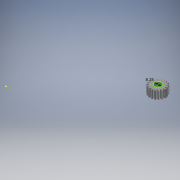
# Autodesk Inventor part: gear_z18_m1
Saved by Autodesk Inventor 2019 (Build 230136000, 136)
## iProperties
Created: 2015-11-26
Part Number: gear_z18_m1
Document SubType Name: Modeling
Designer: VozarikL
Material: Generic
Density: 1 g/cm^3
Appearance: Aluminum - Polished
Autodesk Inventor part; units mm, degrees
ref_plane "YZ Plane" through (0, 0, 0) normal (1, 0, 0) x (0, 1, 0)
ref_plane "XZ Plane" through (0, 0, 0) normal (0, 1, 0) x (-1, 0, 0)
ref_plane "XY Plane" through (0, 0, 0) normal (0, 0, 1) x (1, 0, 0)
sketch "Vázlat1" plane through (0, 0, 0) normal (0, 0, 1) x (1, 0, 0)
  arc A0 (98.9683, 94.0647) -> (99.0231, 94.4245) centre (91.2444, 95.4266) ccw
  arc A1 (99.2517, 94.6057) -> (99.0231, 94.4245) centre (99.2304, 94.3977) ccw
  line L0 (99.2517, 94.6057) -> (99.6575, 94.564)
  line L1 (99.6575, 94.564) -> (99.6743, 94.563)
  line L2 (99.6743, 94.563) -> (99.7248, 94.5628)
  line L3 (99.7248, 94.5628) -> (99.8089, 94.5677)
  line L4 (99.8089, 94.5677) -> (99.9258, 94.5818)
  line L5 (99.9258, 94.5818) -> (100.0748, 94.6094)
  line L6 (100.0748, 94.6094) -> (100.2544, 94.6544)
  line L7 (100.2544, 94.6544) -> (100.4629, 94.7209)
  line L8 (100.4629, 94.7209) -> (100.6981, 94.8126)
  line L9 (100.6981, 94.8126) -> (100.9576, 94.9332)
  line L10 (100.9576, 94.9332) -> (101.2386, 95.0859)
  arc A2 (101.2386, 95.0859) -> (101.2444, 95.4266) centre (91.2444, 95.4266) ccw
  arc A3 (99.0231, 96.4288) -> (98.9683, 96.7885) centre (91.2444, 95.4266) ccw
  arc A4 (99.0231, 96.4288) -> (99.2517, 96.2476) centre (99.2304, 96.4555) ccw
  line L11 (99.2517, 96.2476) -> (99.6575, 96.2892)
  line L12 (99.6575, 96.2892) -> (99.6743, 96.2902)
  line L13 (99.6743, 96.2902) -> (99.7248, 96.2904)
  line L14 (99.7248, 96.2904) -> (99.8089, 96.2856)
  line L15 (99.8089, 96.2856) -> (99.9258, 96.2714)
  line L16 (99.9258, 96.2714) -> (100.0748, 96.2439)
  line L17 (100.0748, 96.2439) -> (100.2544, 96.1988)
  line L18 (100.2544, 96.1988) -> (100.4629, 96.1323)
  line L19 (100.4629, 96.1323) -> (100.6981, 96.0406)
  line L20 (100.6981, 96.0406) -> (100.9576, 95.9201)
  line L21 (100.9576, 95.9201) -> (101.2386, 95.7674)
  arc A5 (101.2444, 95.4266) -> (101.2386, 95.7674) centre (91.2444, 95.4266) ccw
  arc A6 (98.9683, 96.7885) -> (98.8968, 97.1454) centre (91.2444, 95.4266) ccw
  arc A7 (99.0496, 97.3938) -> (98.8968, 97.1454) centre (99.1007, 97.1912) ccw
  line L22 (99.0496, 97.3938) -> (99.4452, 97.4935)
  line L23 (99.4452, 97.4935) -> (99.4613, 97.4983)
  line L24 (99.4613, 97.4983) -> (99.5088, 97.5154)
  line L25 (99.5088, 97.5154) -> (99.5861, 97.5487)
  line L26 (99.5861, 97.5487) -> (99.6912, 97.602)
  line L27 (99.6912, 97.602) -> (99.8218, 97.6788)
  line L28 (99.8218, 97.6788) -> (99.9751, 97.7826)
  line L29 (99.9751, 97.7826) -> (100.1483, 97.9164)
  line L30 (100.1483, 97.9164) -> (100.338, 98.083)
  line L31 (100.338, 98.083) -> (100.5406, 98.285)
  line L32 (100.5406, 98.285) -> (100.7524, 98.5246)
  arc A8 (100.7524, 98.5246) -> (100.6413, 98.8468) centre (91.2444, 95.4266) ccw
  arc A9 (98.2112, 99.0288) -> (98.0366, 99.3481) centre (91.2444, 95.4266) ccw
  arc A10 (98.2112, 99.0288) -> (98.488, 98.9368) centre (98.3969, 99.1248) ccw
  line L33 (98.488, 98.9368) -> (98.8551, 99.1146)
  line L34 (98.8551, 99.1146) -> (98.8706, 99.1213)
  line L35 (98.8706, 99.1213) -> (98.918, 99.1388)
  line L36 (98.918, 99.1388) -> (98.9986, 99.163)
  line L37 (98.9986, 99.163) -> (99.1133, 99.1897)
  line L38 (99.1133, 99.1897) -> (99.2627, 99.2148)
  line L39 (99.2627, 99.2148) -> (99.4469, 99.2339)
  line L40 (99.4469, 99.2339) -> (99.6655, 99.2427)
  line L41 (99.6655, 99.2427) -> (99.918, 99.2369)
  line L42 (99.918, 99.2369) -> (100.2031, 99.2124)
  line L43 (100.2031, 99.2124) -> (100.5193, 99.1651)
  arc A11 (100.6413, 98.8468) -> (100.5193, 99.1651) centre (91.2444, 95.4266) ccw
  arc A12 (98.0366, 99.3481) -> (97.8474, 99.659) centre (91.2444, 95.4266) ccw
  arc A13 (97.9061, 99.9447) -> (97.8474, 99.659) centre (98.0234, 99.7718) ccw
  line L44 (97.9061, 99.9447) -> (98.2437, 100.1737)
  line L45 (98.2437, 100.1737) -> (98.2572, 100.1837)
  line L46 (98.2572, 100.1837) -> (98.296, 100.216)
  line L47 (98.296, 100.216) -> (98.3573, 100.2738)
  line L48 (98.3573, 100.2738) -> (98.4378, 100.3598)
  line L49 (98.4378, 100.3598) -> (98.5342, 100.4766)
  line L50 (98.5342, 100.4766) -> (98.6428, 100.6266)
  line L51 (98.6428, 100.6266) -> (98.7598, 100.8115)
  line L52 (98.7598, 100.8115) -> (98.881, 101.033)
  line L53 (98.881, 101.033) -> (99.0023, 101.2921)
  line L54 (99.0023, 101.2921) -> (99.1194, 101.5897)
  arc A14 (99.1194, 101.5897) -> (98.9049, 101.8545) centre (91.2444, 95.4266) ccw
  arc A15 (96.5591, 101.1944) -> (96.2858, 101.4347) centre (91.2444, 95.4266) ccw
  arc A16 (96.5591, 101.1944) -> (96.8507, 101.2025) centre (96.7007, 101.3481) ccw
  line L55 (96.8507, 101.2025) -> (97.1348, 101.4953)
  line L56 (97.1348, 101.4953) -> (97.147, 101.5068)
  line L57 (97.147, 101.5068) -> (97.1856, 101.5394)
  line L58 (97.1856, 101.5394) -> (97.253, 101.5897)
  line L59 (97.253, 101.5897) -> (97.3517, 101.6541)
  line L60 (97.3517, 101.6541) -> (97.4836, 101.7287)
  line L61 (97.4836, 101.7287) -> (97.6501, 101.8097)
  line L62 (97.6501, 101.8097) -> (97.8525, 101.8927)
  line L63 (97.8525, 101.8927) -> (98.0917, 101.9737)
  line L64 (98.0917, 101.9737) -> (98.368, 102.0482)
  line L65 (98.368, 102.0482) -> (98.6814, 102.1118)
  arc A17 (98.9049, 101.8545) -> (98.6814, 102.1118) centre (91.2444, 95.4266) ccw
  arc A18 (96.2858, 101.4347) -> (96.0017, 101.6621) centre (91.2444, 95.4266) ccw
  arc A19 (95.959, 101.9507) -> (96.0017, 101.6621) centre (96.1284, 101.8283) ccw
  line L66 (95.959, 101.9507) -> (96.198, 102.2813)
  line L67 (96.198, 102.2813) -> (96.2073, 102.2954)
  line L68 (96.2073, 102.2954) -> (96.2327, 102.339)
  line L69 (96.2327, 102.339) -> (96.2705, 102.4142)
  line L70 (96.2705, 102.4142) -> (96.3168, 102.5226)
  line L71 (96.3168, 102.5226) -> (96.3674, 102.6653)
  line L72 (96.3674, 102.6653) -> (96.4181, 102.8434)
  line L73 (96.4181, 102.8434) -> (96.4648, 103.0572)
  line L74 (96.4648, 103.0572) -> (96.503, 103.3068)
  line L75 (96.503, 103.3068) -> (96.5284, 103.5918)
  line L76 (96.5284, 103.5918) -> (96.5366, 103.9115)
  arc A20 (96.5366, 103.9115) -> (96.2444, 104.0869) centre (91.2444, 95.4266) ccw
  arc A21 (94.2659, 102.6643) -> (93.9269, 102.7966) centre (91.2444, 95.4266) ccw
  arc A22 (94.2659, 102.6643) -> (94.5371, 102.7716) centre (94.3464, 102.8571) ccw
  line L77 (94.5371, 102.7716) -> (94.704, 103.1439)
  line L78 (94.704, 103.1439) -> (94.7115, 103.159)
  line L79 (94.7115, 103.159) -> (94.7366, 103.2028)
  line L80 (94.7366, 103.2028) -> (94.7828, 103.2731)
  line L81 (94.7828, 103.2731) -> (94.8535, 103.3674)
  line L82 (94.8535, 103.3674) -> (94.9518, 103.4826)
  line L83 (94.9518, 103.4826) -> (95.0806, 103.6156)
  line L84 (95.0806, 103.6156) -> (95.2425, 103.7629)
  line L85 (95.2425, 103.7629) -> (95.4395, 103.9207)
  line L86 (95.4395, 103.9207) -> (95.6737, 104.0852)
  line L87 (95.6737, 104.0852) -> (95.9464, 104.2522)
  arc A23 (96.2444, 104.0869) -> (95.9464, 104.2522) centre (91.2444, 95.4266) ccw
  arc A24 (93.9269, 102.7966) -> (93.5821, 102.9131) centre (91.2444, 95.4266) ccw
  arc A25 (93.4434, 103.1697) -> (93.5821, 102.9131) centre (93.6444, 103.1126) ccw
  line L88 (93.4434, 103.1697) -> (93.5548, 103.5622)
  line L89 (93.5548, 103.5622) -> (93.5587, 103.5785)
  line L90 (93.5587, 103.5785) -> (93.5677, 103.6282)
  line L91 (93.5677, 103.6282) -> (93.5775, 103.7118)
  line L92 (93.5775, 103.7118) -> (93.5839, 103.8295)
  line L93 (93.5839, 103.8295) -> (93.5826, 103.9809)
  line L94 (93.5826, 103.9809) -> (93.5694, 104.1656)
  line L95 (93.5694, 104.1656) -> (93.5402, 104.3825)
  line L96 (93.5402, 104.3825) -> (93.4907, 104.6301)
  line L97 (93.4907, 104.6301) -> (93.4171, 104.9066)
  line L98 (93.4171, 104.9066) -> (93.3155, 105.2098)
  arc A26 (93.3155, 105.2098) -> (92.9809, 105.2747) centre (91.2444, 95.4266) ccw
  arc A27 (91.6082, 103.2612) -> (91.2444, 103.2696) centre (91.2444, 95.4266) ccw
  arc A28 (91.6082, 103.2612) -> (91.8264, 103.4548) centre (91.6179, 103.47) ccw
  line L99 (91.8264, 103.4548) -> (91.8559, 103.8617)
  line L100 (91.8559, 103.8617) -> (91.8578, 103.8785)
  line L101 (91.8578, 103.8785) -> (91.8664, 103.9282)
  line L102 (91.8664, 103.9282) -> (91.8857, 104.0101)
  line L103 (91.8857, 104.0101) -> (91.9199, 104.1229)
  line L104 (91.9199, 104.1229) -> (91.9729, 104.2648)
  line L105 (91.9729, 104.2648) -> (92.0485, 104.4338)
  line L106 (92.0485, 104.4338) -> (92.1502, 104.6276)
  line L107 (92.1502, 104.6276) -> (92.2814, 104.8433)
  line L108 (92.2814, 104.8433) -> (92.4451, 105.0779)
  line L109 (92.4451, 105.0779) -> (92.6443, 105.3282)
  arc A29 (92.9809, 105.2747) -> (92.6443, 105.3282) centre (91.2444, 95.4266) ccw
  arc A30 (91.2444, 103.2696) -> (90.8806, 103.2612) centre (91.2444, 95.4266) ccw
  arc A31 (90.6625, 103.4548) -> (90.8806, 103.2612) centre (90.8709, 103.47) ccw
  line L110 (90.6625, 103.4548) -> (90.633, 103.8617)
  line L111 (90.633, 103.8617) -> (90.631, 103.8785)
  line L112 (90.631, 103.8785) -> (90.6225, 103.9282)
  line L113 (90.6225, 103.9282) -> (90.6031, 104.0101)
  line L114 (90.6031, 104.0101) -> (90.5689, 104.1229)
  line L115 (90.5689, 104.1229) -> (90.5159, 104.2648)
  line L116 (90.5159, 104.2648) -> (90.4403, 104.4338)
  line L117 (90.4403, 104.4338) -> (90.3386, 104.6276)
  line L118 (90.3386, 104.6276) -> (90.2075, 104.8433)
  line L119 (90.2075, 104.8433) -> (90.0437, 105.0779)
  line L120 (90.0437, 105.0779) -> (89.8445, 105.3282)
  arc A32 (89.8445, 105.3282) -> (89.5079, 105.2747) centre (91.2444, 95.4266) ccw
  arc A33 (88.9067, 102.9131) -> (88.5619, 102.7966) centre (91.2444, 95.4266) ccw
  arc A34 (88.9067, 102.9131) -> (89.0455, 103.1697) centre (88.8444, 103.1126) ccw
  line L121 (89.0455, 103.1697) -> (88.934, 103.5622)
  line L122 (88.934, 103.5622) -> (88.9301, 103.5785)
  line L123 (88.9301, 103.5785) -> (88.9211, 103.6282)
  line L124 (88.9211, 103.6282) -> (88.9113, 103.7118)
  line L125 (88.9113, 103.7118) -> (88.9049, 103.8295)
  line L126 (88.9049, 103.8295) -> (88.9062, 103.9809)
  line L127 (88.9062, 103.9809) -> (88.9194, 104.1656)
  line L128 (88.9194, 104.1656) -> (88.9487, 104.3825)
  line L129 (88.9487, 104.3825) -> (88.9981, 104.6301)
  line L130 (88.9981, 104.6301) -> (89.0718, 104.9066)
  line L131 (89.0718, 104.9066) -> (89.1733, 105.2098)
  arc A35 (89.5079, 105.2747) -> (89.1733, 105.2098) centre (91.2444, 95.4266) ccw
  arc A36 (88.5619, 102.7966) -> (88.223, 102.6643) centre (91.2444, 95.4266) ccw
  arc A37 (87.9517, 102.7716) -> (88.223, 102.6643) centre (88.1425, 102.8571) ccw
  line L132 (87.9517, 102.7716) -> (87.7849, 103.1439)
  line L133 (87.7849, 103.1439) -> (87.7773, 103.159)
  line L134 (87.7773, 103.159) -> (87.7523, 103.2028)
  line L135 (87.7523, 103.2028) -> (87.7061, 103.2731)
  line L136 (87.7061, 103.2731) -> (87.6353, 103.3674)
  line L137 (87.6353, 103.3674) -> (87.537, 103.4826)
  line L138 (87.537, 103.4826) -> (87.4082, 103.6156)
  line L139 (87.4082, 103.6156) -> (87.2464, 103.7629)
  line L140 (87.2464, 103.7629) -> (87.0493, 103.9207)
  line L141 (87.0493, 103.9207) -> (86.8152, 104.0852)
  line L142 (86.8152, 104.0852) -> (86.5424, 104.2522)
  arc A38 (86.5424, 104.2522) -> (86.2444, 104.0869) centre (91.2444, 95.4266) ccw
  arc A39 (86.4871, 101.6621) -> (86.203, 101.4347) centre (91.2444, 95.4266) ccw
  arc A40 (86.4871, 101.6621) -> (86.5298, 101.9507) centre (86.3604, 101.8283) ccw
  line L143 (86.5298, 101.9507) -> (86.2908, 102.2813)
  line L144 (86.2908, 102.2813) -> (86.2816, 102.2954)
  line L145 (86.2816, 102.2954) -> (86.2561, 102.339)
  line L146 (86.2561, 102.339) -> (86.2183, 102.4142)
  line L147 (86.2183, 102.4142) -> (86.1721, 102.5226)
  line L148 (86.1721, 102.5226) -> (86.1215, 102.6653)
  line L149 (86.1215, 102.6653) -> (86.0707, 102.8434)
  line L150 (86.0707, 102.8434) -> (86.024, 103.0572)
  line L151 (86.024, 103.0572) -> (85.9858, 103.3068)
  line L152 (85.9858, 103.3068) -> (85.9605, 103.5918)
  line L153 (85.9605, 103.5918) -> (85.9522, 103.9115)
  arc A41 (86.2444, 104.0869) -> (85.9522, 103.9115) centre (91.2444, 95.4266) ccw
  arc A42 (86.203, 101.4347) -> (85.9298, 101.1944) centre (91.2444, 95.4266) ccw
  arc A43 (85.6382, 101.2025) -> (85.9298, 101.1944) centre (85.7881, 101.3481) ccw
  line L154 (85.6382, 101.2025) -> (85.354, 101.4953)
  line L155 (85.354, 101.4953) -> (85.3418, 101.5068)
  line L156 (85.3418, 101.5068) -> (85.3033, 101.5394)
  line L157 (85.3033, 101.5394) -> (85.2358, 101.5897)
  line L158 (85.2358, 101.5897) -> (85.1371, 101.6541)
  line L159 (85.1371, 101.6541) -> (85.0053, 101.7287)
  line L160 (85.0053, 101.7287) -> (84.8387, 101.8097)
  line L161 (84.8387, 101.8097) -> (84.6363, 101.8927)
  line L162 (84.6363, 101.8927) -> (84.3971, 101.9737)
  line L163 (84.3971, 101.9737) -> (84.1209, 102.0482)
  line L164 (84.1209, 102.0482) -> (83.8075, 102.1118)
  arc A44 (83.8075, 102.1118) -> (83.584, 101.8545) centre (91.2444, 95.4266) ccw
  arc A45 (84.6414, 99.659) -> (84.4522, 99.3481) centre (91.2444, 95.4266) ccw
  arc A46 (84.6414, 99.659) -> (84.5827, 99.9447) centre (84.4654, 99.7718) ccw
  line L165 (84.5827, 99.9447) -> (84.2451, 100.1737)
  line L166 (84.2451, 100.1737) -> (84.2316, 100.1837)
  line L167 (84.2316, 100.1837) -> (84.1928, 100.216)
  line L168 (84.1928, 100.216) -> (84.1315, 100.2738)
  line L169 (84.1315, 100.2738) -> (84.051, 100.3598)
  line L170 (84.051, 100.3598) -> (83.9546, 100.4766)
  line L171 (83.9546, 100.4766) -> (83.846, 100.6266)
  line L172 (83.846, 100.6266) -> (83.7291, 100.8115)
  line L173 (83.7291, 100.8115) -> (83.6078, 101.033)
  line L174 (83.6078, 101.033) -> (83.4865, 101.2921)
  line L175 (83.4865, 101.2921) -> (83.3694, 101.5897)
  arc A47 (83.584, 101.8545) -> (83.3694, 101.5897) centre (91.2444, 95.4266) ccw
  arc A48 (84.4522, 99.3481) -> (84.2776, 99.0288) centre (91.2444, 95.4266) ccw
  arc A49 (84.0008, 98.9368) -> (84.2776, 99.0288) centre (84.0919, 99.1248) ccw
  line L176 (84.0008, 98.9368) -> (83.6337, 99.1146)
  line L177 (83.6337, 99.1146) -> (83.6182, 99.1213)
  line L178 (83.6182, 99.1213) -> (83.5709, 99.1388)
  line L179 (83.5709, 99.1388) -> (83.4902, 99.163)
  line L180 (83.4902, 99.163) -> (83.3755, 99.1897)
  line L181 (83.3755, 99.1897) -> (83.2261, 99.2148)
  line L182 (83.2261, 99.2148) -> (83.0419, 99.2339)
  line L183 (83.0419, 99.2339) -> (82.8233, 99.2427)
  line L184 (82.8233, 99.2427) -> (82.5709, 99.2369)
  line L185 (82.5709, 99.2369) -> (82.2858, 99.2124)
  line L186 (82.2858, 99.2124) -> (81.9695, 99.1651)
  arc A50 (81.9695, 99.1651) -> (81.8475, 98.8468) centre (91.2444, 95.4266) ccw
  arc A51 (83.5921, 97.1454) -> (83.5206, 96.7885) centre (91.2444, 95.4266) ccw
  arc A52 (83.5921, 97.1454) -> (83.4392, 97.3938) centre (83.3881, 97.1912) ccw
  line L187 (83.4392, 97.3938) -> (83.0436, 97.4935)
  line L188 (83.0436, 97.4935) -> (83.0275, 97.4983)
  line L189 (83.0275, 97.4983) -> (82.98, 97.5154)
  line L190 (82.98, 97.5154) -> (82.9027, 97.5487)
  line L191 (82.9027, 97.5487) -> (82.7976, 97.602)
  line L192 (82.7976, 97.602) -> (82.667, 97.6788)
  line L193 (82.667, 97.6788) -> (82.5137, 97.7826)
  line L194 (82.5137, 97.7826) -> (82.3405, 97.9164)
  line L195 (82.3405, 97.9164) -> (82.1509, 98.083)
  line L196 (82.1509, 98.083) -> (81.9482, 98.285)
  line L197 (81.9482, 98.285) -> (81.7364, 98.5246)
  arc A53 (81.8475, 98.8468) -> (81.7364, 98.5246) centre (91.2444, 95.4266) ccw
  arc A54 (83.5206, 96.7885) -> (83.4657, 96.4288) centre (91.2444, 95.4266) ccw
  arc A55 (83.2371, 96.2476) -> (83.4657, 96.4288) centre (83.2584, 96.4555) ccw
  line L198 (83.2371, 96.2476) -> (82.8313, 96.2892)
  line L199 (82.8313, 96.2892) -> (82.8145, 96.2902)
  line L200 (82.8145, 96.2902) -> (82.764, 96.2904)
  line L201 (82.764, 96.2904) -> (82.68, 96.2856)
  line L202 (82.68, 96.2856) -> (82.563, 96.2714)
  line L203 (82.563, 96.2714) -> (82.414, 96.2439)
  line L204 (82.414, 96.2439) -> (82.2344, 96.1988)
  line L205 (82.2344, 96.1988) -> (82.026, 96.1323)
  line L206 (82.026, 96.1323) -> (81.7907, 96.0406)
  line L207 (81.7907, 96.0406) -> (81.5312, 95.9201)
  line L208 (81.5312, 95.9201) -> (81.2502, 95.7674)
  arc A56 (81.2502, 95.7674) -> (81.2444, 95.4266) centre (91.2444, 95.4266) ccw
  arc A57 (83.4657, 94.4245) -> (83.5206, 94.0647) centre (91.2444, 95.4266) ccw
  arc A58 (83.4657, 94.4245) -> (83.2371, 94.6057) centre (83.2584, 94.3977) ccw
  line L209 (83.2371, 94.6057) -> (82.8313, 94.564)
  line L210 (82.8313, 94.564) -> (82.8145, 94.563)
  line L211 (82.8145, 94.563) -> (82.764, 94.5628)
  line L212 (82.764, 94.5628) -> (82.68, 94.5677)
  line L213 (82.68, 94.5677) -> (82.563, 94.5818)
  line L214 (82.563, 94.5818) -> (82.414, 94.6094)
  line L215 (82.414, 94.6094) -> (82.2344, 94.6544)
  line L216 (82.2344, 94.6544) -> (82.026, 94.7209)
  line L217 (82.026, 94.7209) -> (81.7907, 94.8126)
  line L218 (81.7907, 94.8126) -> (81.5312, 94.9332)
  line L219 (81.5312, 94.9332) -> (81.2502, 95.0859)
  arc A59 (81.2444, 95.4266) -> (81.2502, 95.0859) centre (91.2444, 95.4266) ccw
  arc A60 (83.5206, 94.0647) -> (83.5921, 93.7079) centre (91.2444, 95.4266) ccw
  arc A61 (83.4392, 93.4594) -> (83.5921, 93.7079) centre (83.3881, 93.6621) ccw
  line L220 (83.4392, 93.4594) -> (83.0436, 93.3597)
  line L221 (83.0436, 93.3597) -> (83.0275, 93.3549)
  line L222 (83.0275, 93.3549) -> (82.98, 93.3379)
  line L223 (82.98, 93.3379) -> (82.9027, 93.3046)
  line L224 (82.9027, 93.3046) -> (82.7976, 93.2513)
  line L225 (82.7976, 93.2513) -> (82.667, 93.1744)
  line L226 (82.667, 93.1744) -> (82.5137, 93.0707)
  line L227 (82.5137, 93.0707) -> (82.3405, 92.9369)
  line L228 (82.3405, 92.9369) -> (82.1509, 92.7702)
  line L229 (82.1509, 92.7702) -> (81.9482, 92.5682)
  line L230 (81.9482, 92.5682) -> (81.7364, 92.3286)
  arc A62 (81.7364, 92.3286) -> (81.8475, 92.0064) centre (91.2444, 95.4266) ccw
  arc A63 (84.2776, 91.8244) -> (84.4522, 91.5051) centre (91.2444, 95.4266) ccw
  arc A64 (84.2776, 91.8244) -> (84.0008, 91.9165) centre (84.0919, 91.7284) ccw
  line L231 (84.0008, 91.9165) -> (83.6337, 91.7386)
  line L232 (83.6337, 91.7386) -> (83.6182, 91.7319)
  line L233 (83.6182, 91.7319) -> (83.5709, 91.7144)
  line L234 (83.5709, 91.7144) -> (83.4902, 91.6903)
  line L235 (83.4902, 91.6903) -> (83.3755, 91.6635)
  line L236 (83.3755, 91.6635) -> (83.2261, 91.6385)
  line L237 (83.2261, 91.6385) -> (83.0419, 91.6194)
  line L238 (83.0419, 91.6194) -> (82.8233, 91.6106)
  line L239 (82.8233, 91.6106) -> (82.5709, 91.6163)
  line L240 (82.5709, 91.6163) -> (82.2858, 91.6408)
  line L241 (82.2858, 91.6408) -> (81.9695, 91.6882)
  arc A65 (81.8475, 92.0064) -> (81.9695, 91.6882) centre (91.2444, 95.4266) ccw
  arc A66 (84.4522, 91.5051) -> (84.6414, 91.1943) centre (91.2444, 95.4266) ccw
  arc A67 (84.5827, 90.9085) -> (84.6414, 91.1943) centre (84.4654, 91.0815) ccw
  line L242 (84.5827, 90.9085) -> (84.2451, 90.6795)
  line L243 (84.2451, 90.6795) -> (84.2316, 90.6695)
  line L244 (84.2316, 90.6695) -> (84.1928, 90.6372)
  line L245 (84.1928, 90.6372) -> (84.1315, 90.5795)
  line L246 (84.1315, 90.5795) -> (84.051, 90.4935)
  line L247 (84.051, 90.4935) -> (83.9546, 90.3766)
  line L248 (83.9546, 90.3766) -> (83.846, 90.2267)
  line L249 (83.846, 90.2267) -> (83.7291, 90.0417)
  line L250 (83.7291, 90.0417) -> (83.6078, 89.8203)
  line L251 (83.6078, 89.8203) -> (83.4865, 89.5611)
  line L252 (83.4865, 89.5611) -> (83.3694, 89.2635)
  arc A68 (83.3694, 89.2635) -> (83.584, 88.9988) centre (91.2444, 95.4266) ccw
  arc A69 (85.9298, 89.6589) -> (86.203, 89.4185) centre (91.2444, 95.4266) ccw
  arc A70 (85.9298, 89.6589) -> (85.6382, 89.6507) centre (85.7881, 89.5052) ccw
  line L253 (85.6382, 89.6507) -> (85.354, 89.358)
  line L254 (85.354, 89.358) -> (85.3418, 89.3464)
  line L255 (85.3418, 89.3464) -> (85.3033, 89.3138)
  line L256 (85.3033, 89.3138) -> (85.2358, 89.2635)
  line L257 (85.2358, 89.2635) -> (85.1371, 89.1991)
  line L258 (85.1371, 89.1991) -> (85.0053, 89.1245)
  line L259 (85.0053, 89.1245) -> (84.8387, 89.0436)
  line L260 (84.8387, 89.0436) -> (84.6363, 88.9605)
  line L261 (84.6363, 88.9605) -> (84.3971, 88.8796)
  line L262 (84.3971, 88.8796) -> (84.1209, 88.8051)
  line L263 (84.1209, 88.8051) -> (83.8075, 88.7414)
  arc A71 (83.584, 88.9988) -> (83.8075, 88.7414) centre (91.2444, 95.4266) ccw
  arc A72 (86.203, 89.4185) -> (86.4871, 89.1912) centre (91.2444, 95.4266) ccw
  arc A73 (86.5298, 88.9026) -> (86.4871, 89.1912) centre (86.3604, 89.025) ccw
  line L264 (86.5298, 88.9026) -> (86.2908, 88.5719)
  line L265 (86.2908, 88.5719) -> (86.2816, 88.5579)
  line L266 (86.2816, 88.5579) -> (86.2561, 88.5143)
  line L267 (86.2561, 88.5143) -> (86.2183, 88.4391)
  line L268 (86.2183, 88.4391) -> (86.1721, 88.3307)
  line L269 (86.1721, 88.3307) -> (86.1215, 88.1879)
  line L270 (86.1215, 88.1879) -> (86.0707, 88.0099)
  line L271 (86.0707, 88.0099) -> (86.024, 87.7961)
  line L272 (86.024, 87.7961) -> (85.9858, 87.5465)
  line L273 (85.9858, 87.5465) -> (85.9605, 87.2615)
  line L274 (85.9605, 87.2615) -> (85.9522, 86.9418)
  arc A74 (85.9522, 86.9418) -> (86.2444, 86.7664) centre (91.2444, 95.4266) ccw
  arc A75 (88.223, 88.189) -> (88.5619, 88.0566) centre (91.2444, 95.4266) ccw
  arc A76 (88.223, 88.189) -> (87.9517, 88.0816) centre (88.1425, 87.9961) ccw
  line L275 (87.9517, 88.0816) -> (87.7849, 87.7094)
  line L276 (87.7849, 87.7094) -> (87.7773, 87.6943)
  line L277 (87.7773, 87.6943) -> (87.7523, 87.6505)
  line L278 (87.7523, 87.6505) -> (87.7061, 87.5801)
  line L279 (87.7061, 87.5801) -> (87.6353, 87.4859)
  line L280 (87.6353, 87.4859) -> (87.537, 87.3707)
  line L281 (87.537, 87.3707) -> (87.4082, 87.2377)
  line L282 (87.4082, 87.2377) -> (87.2464, 87.0904)
  line L283 (87.2464, 87.0904) -> (87.0493, 86.9325)
  line L284 (87.0493, 86.9325) -> (86.8152, 86.768)
  line L285 (86.8152, 86.768) -> (86.5424, 86.601)
  arc A77 (86.2444, 86.7664) -> (86.5424, 86.601) centre (91.2444, 95.4266) ccw
  arc A78 (88.5619, 88.0566) -> (88.9067, 87.9401) centre (91.2444, 95.4266) ccw
  arc A79 (89.0455, 87.6835) -> (88.9067, 87.9401) centre (88.8444, 87.7406) ccw
  line L286 (89.0455, 87.6835) -> (88.934, 87.2911)
  line L287 (88.934, 87.2911) -> (88.9301, 87.2747)
  line L288 (88.9301, 87.2747) -> (88.9211, 87.225)
  line L289 (88.9211, 87.225) -> (88.9113, 87.1414)
  line L290 (88.9113, 87.1414) -> (88.9049, 87.0238)
  line L291 (88.9049, 87.0238) -> (88.9062, 86.8723)
  line L292 (88.9062, 86.8723) -> (88.9194, 86.6876)
  line L293 (88.9194, 86.6876) -> (88.9487, 86.4708)
  line L294 (88.9487, 86.4708) -> (88.9981, 86.2232)
  line L295 (88.9981, 86.2232) -> (89.0718, 85.9467)
  line L296 (89.0718, 85.9467) -> (89.1733, 85.6434)
  arc A80 (89.1733, 85.6434) -> (89.5079, 85.5785) centre (91.2444, 95.4266) ccw
  arc A81 (90.8806, 87.5921) -> (91.2444, 87.5836) centre (91.2444, 95.4266) ccw
  arc A82 (90.8806, 87.5921) -> (90.6625, 87.3984) centre (90.8709, 87.3833) ccw
  line L297 (90.6625, 87.3984) -> (90.633, 86.9915)
  line L298 (90.633, 86.9915) -> (90.631, 86.9748)
  line L299 (90.631, 86.9748) -> (90.6225, 86.925)
  line L300 (90.6225, 86.925) -> (90.6031, 86.8431)
  line L301 (90.6031, 86.8431) -> (90.5689, 86.7304)
  line L302 (90.5689, 86.7304) -> (90.5159, 86.5885)
  line L303 (90.5159, 86.5885) -> (90.4403, 86.4194)
  line L304 (90.4403, 86.4194) -> (90.3386, 86.2257)
  line L305 (90.3386, 86.2257) -> (90.2075, 86.01)
  line L306 (90.2075, 86.01) -> (90.0437, 85.7753)
  line L307 (90.0437, 85.7753) -> (89.8445, 85.5251)
  arc A83 (89.5079, 85.5785) -> (89.8445, 85.5251) centre (91.2444, 95.4266) ccw
  arc A84 (91.2444, 87.5836) -> (91.6082, 87.5921) centre (91.2444, 95.4266) ccw
  arc A85 (91.8264, 87.3984) -> (91.6082, 87.5921) centre (91.6179, 87.3833) ccw
  line L308 (91.8264, 87.3984) -> (91.8559, 86.9915)
  line L309 (91.8559, 86.9915) -> (91.8578, 86.9748)
  line L310 (91.8578, 86.9748) -> (91.8664, 86.925)
  line L311 (91.8664, 86.925) -> (91.8857, 86.8431)
  line L312 (91.8857, 86.8431) -> (91.9199, 86.7304)
  line L313 (91.9199, 86.7304) -> (91.9729, 86.5885)
  line L314 (91.9729, 86.5885) -> (92.0485, 86.4194)
  line L315 (92.0485, 86.4194) -> (92.1502, 86.2257)
  line L316 (92.1502, 86.2257) -> (92.2814, 86.01)
  line L317 (92.2814, 86.01) -> (92.4451, 85.7753)
  line L318 (92.4451, 85.7753) -> (92.6443, 85.5251)
  arc A86 (92.6443, 85.5251) -> (92.9809, 85.5785) centre (91.2444, 95.4266) ccw
  arc A87 (93.5821, 87.9401) -> (93.9269, 88.0566) centre (91.2444, 95.4266) ccw
  arc A88 (93.5821, 87.9401) -> (93.4434, 87.6835) centre (93.6444, 87.7406) ccw
  line L319 (93.4434, 87.6835) -> (93.5548, 87.2911)
  line L320 (93.5548, 87.2911) -> (93.5587, 87.2747)
  line L321 (93.5587, 87.2747) -> (93.5677, 87.225)
  line L322 (93.5677, 87.225) -> (93.5775, 87.1414)
  line L323 (93.5775, 87.1414) -> (93.5839, 87.0238)
  line L324 (93.5839, 87.0238) -> (93.5826, 86.8723)
  line L325 (93.5826, 86.8723) -> (93.5694, 86.6876)
  line L326 (93.5694, 86.6876) -> (93.5402, 86.4708)
  line L327 (93.5402, 86.4708) -> (93.4907, 86.2232)
  line L328 (93.4907, 86.2232) -> (93.4171, 85.9467)
  line L329 (93.4171, 85.9467) -> (93.3155, 85.6434)
  arc A89 (92.9809, 85.5785) -> (93.3155, 85.6434) centre (91.2444, 95.4266) ccw
  arc A90 (93.9269, 88.0566) -> (94.2659, 88.189) centre (91.2444, 95.4266) ccw
  arc A91 (94.5371, 88.0816) -> (94.2659, 88.189) centre (94.3464, 87.9961) ccw
  line L330 (94.5371, 88.0816) -> (94.704, 87.7094)
  line L331 (94.704, 87.7094) -> (94.7115, 87.6943)
  line L332 (94.7115, 87.6943) -> (94.7366, 87.6505)
  line L333 (94.7366, 87.6505) -> (94.7828, 87.5801)
  line L334 (94.7828, 87.5801) -> (94.8535, 87.4859)
  line L335 (94.8535, 87.4859) -> (94.9518, 87.3707)
  line L336 (94.9518, 87.3707) -> (95.0806, 87.2377)
  line L337 (95.0806, 87.2377) -> (95.2425, 87.0904)
  line L338 (95.2425, 87.0904) -> (95.4395, 86.9325)
  line L339 (95.4395, 86.9325) -> (95.6737, 86.768)
  line L340 (95.6737, 86.768) -> (95.9464, 86.601)
  arc A92 (95.9464, 86.601) -> (96.2444, 86.7664) centre (91.2444, 95.4266) ccw
  arc A93 (96.0017, 89.1912) -> (96.2858, 89.4185) centre (91.2444, 95.4266) ccw
  arc A94 (96.0017, 89.1912) -> (95.959, 88.9026) centre (96.1284, 89.025) ccw
  line L341 (95.959, 88.9026) -> (96.198, 88.5719)
  line L342 (96.198, 88.5719) -> (96.2073, 88.5579)
  line L343 (96.2073, 88.5579) -> (96.2327, 88.5143)
  line L344 (96.2327, 88.5143) -> (96.2705, 88.4391)
  line L345 (96.2705, 88.4391) -> (96.3168, 88.3307)
  line L346 (96.3168, 88.3307) -> (96.3674, 88.1879)
  line L347 (96.3674, 88.1879) -> (96.4181, 88.0099)
  line L348 (96.4181, 88.0099) -> (96.4648, 87.7961)
  line L349 (96.4648, 87.7961) -> (96.503, 87.5465)
  line L350 (96.503, 87.5465) -> (96.5284, 87.2615)
  line L351 (96.5284, 87.2615) -> (96.5366, 86.9418)
  arc A95 (96.2444, 86.7664) -> (96.5366, 86.9418) centre (91.2444, 95.4266) ccw
  arc A96 (96.2858, 89.4185) -> (96.5591, 89.6589) centre (91.2444, 95.4266) ccw
  arc A97 (96.8507, 89.6507) -> (96.5591, 89.6589) centre (96.7007, 89.5052) ccw
  line L352 (96.8507, 89.6507) -> (97.1348, 89.358)
  line L353 (97.1348, 89.358) -> (97.147, 89.3464)
  line L354 (97.147, 89.3464) -> (97.1856, 89.3138)
  line L355 (97.1856, 89.3138) -> (97.253, 89.2635)
  line L356 (97.253, 89.2635) -> (97.3517, 89.1991)
  line L357 (97.3517, 89.1991) -> (97.4836, 89.1245)
  line L358 (97.4836, 89.1245) -> (97.6501, 89.0436)
  line L359 (97.6501, 89.0436) -> (97.8525, 88.9605)
  line L360 (97.8525, 88.9605) -> (98.0917, 88.8796)
  line L361 (98.0917, 88.8796) -> (98.368, 88.8051)
  line L362 (98.368, 88.8051) -> (98.6814, 88.7414)
  arc A98 (98.6814, 88.7414) -> (98.9049, 88.9988) centre (91.2444, 95.4266) ccw
  arc A99 (97.8474, 91.1943) -> (98.0366, 91.5051) centre (91.2444, 95.4266) ccw
  arc A100 (97.8474, 91.1943) -> (97.9061, 90.9085) centre (98.0234, 91.0815) ccw
  line L363 (97.9061, 90.9085) -> (98.2437, 90.6795)
  line L364 (98.2437, 90.6795) -> (98.2572, 90.6695)
  line L365 (98.2572, 90.6695) -> (98.296, 90.6372)
  line L366 (98.296, 90.6372) -> (98.3573, 90.5795)
  line L367 (98.3573, 90.5795) -> (98.4378, 90.4935)
  line L368 (98.4378, 90.4935) -> (98.5342, 90.3766)
  line L369 (98.5342, 90.3766) -> (98.6428, 90.2267)
  line L370 (98.6428, 90.2267) -> (98.7598, 90.0417)
  line L371 (98.7598, 90.0417) -> (98.881, 89.8203)
  line L372 (98.881, 89.8203) -> (99.0023, 89.5611)
  line L373 (99.0023, 89.5611) -> (99.1194, 89.2635)
  arc A101 (98.9049, 88.9988) -> (99.1194, 89.2635) centre (91.2444, 95.4266) ccw
  arc A102 (98.0366, 91.5051) -> (98.2112, 91.8244) centre (91.2444, 95.4266) ccw
  arc A103 (98.488, 91.9165) -> (98.2112, 91.8244) centre (98.3969, 91.7284) ccw
  line L374 (98.488, 91.9165) -> (98.8551, 91.7386)
  line L375 (98.8551, 91.7386) -> (98.8706, 91.7319)
  line L376 (98.8706, 91.7319) -> (98.918, 91.7144)
  line L377 (98.918, 91.7144) -> (98.9986, 91.6903)
  line L378 (98.9986, 91.6903) -> (99.1133, 91.6635)
  line L379 (99.1133, 91.6635) -> (99.2627, 91.6385)
  line L380 (99.2627, 91.6385) -> (99.4469, 91.6194)
  line L381 (99.4469, 91.6194) -> (99.6655, 91.6106)
  line L382 (99.6655, 91.6106) -> (99.918, 91.6163)
  line L383 (99.918, 91.6163) -> (100.2031, 91.6408)
  line L384 (100.2031, 91.6408) -> (100.5193, 91.6882)
  arc A104 (100.5193, 91.6882) -> (100.6413, 92.0064) centre (91.2444, 95.4266) ccw
  arc A105 (98.8968, 93.7079) -> (98.9683, 94.0647) centre (91.2444, 95.4266) ccw
  arc A106 (98.8968, 93.7079) -> (99.0496, 93.4594) centre (99.1007, 93.6621) ccw
  line L385 (99.0496, 93.4594) -> (99.4452, 93.3597)
  line L386 (99.4452, 93.3597) -> (99.4613, 93.3549)
  line L387 (99.4613, 93.3549) -> (99.5088, 93.3379)
  line L388 (99.5088, 93.3379) -> (99.5861, 93.3046)
  line L389 (99.5861, 93.3046) -> (99.6912, 93.2513)
  line L390 (99.6912, 93.2513) -> (99.8218, 93.1744)
  line L391 (99.8218, 93.1744) -> (99.9751, 93.0707)
  line L392 (99.9751, 93.0707) -> (100.1483, 92.9369)
  line L393 (100.1483, 92.9369) -> (100.338, 92.7702)
  line L394 (100.338, 92.7702) -> (100.5406, 92.5682)
  line L395 (100.5406, 92.5682) -> (100.7524, 92.3286)
  arc A107 (100.6413, 92.0064) -> (100.7524, 92.3286) centre (91.2444, 95.4266) ccw
  constraints: 792 end point, 216 point on circle, 108 centre point
extrude "Kihúzás2" add sketch "Vázlat1" along normal blind 10
fillet "Lekerekítés1" radius 0.4 18 edges at (86.3927, 104.1708, 10) (83.6946, 101.9841, 10) (89.676, 105.3029, 10) (93.1485, 105.2437, 10) (96.3913, 104.0004, 10) (99.0133, 101.723, 10) (81.9071, 99.0065, 10) (81.2459, 95.597, 10) (81.7906, 92.1671, 10) (83.4755, 89.1302, 10) (86.0976, 86.8528, 10) (89.3404, 85.6096, 10) (92.8128, 85.5504, 10) (96.0961, 86.6824, 10) (98.7942, 88.8691, 10) (100.5817, 91.8468, 10) (101.243, 95.2562, 10) (100.6983, 98.6862, 10)
fillet "Lekerekítés2" radius 0.4 18 edges at (93.1485, 105.2437, 0) (89.676, 105.3029, 0) (86.3927, 104.1708, 0) (83.6946, 101.9841, 0) (81.9071, 99.0065, 0) (81.2459, 95.597, 0) (81.7906, 92.1671, 0) (101.243, 95.2562, 0) (100.6983, 98.6862, 0) (100.5817, 91.8468, 0) (98.7942, 88.8691, 0) (96.0961, 86.6824, 0) (92.8128, 85.5504, 0) (89.3404, 85.6096, 0) (86.0976, 86.8528, 0) (83.4755, 89.1302, 0) (99.0133, 101.723, 0) (96.3913, 104.0004, 0)
sketch "Vázlat2" plane through (0, 0, 0) normal (0, 0, -1) x (-1, 0, 0)
  arc A0 (-98.8968, 97.1454) -> (-99.0231, 96.4288) centre (-91.2444, 95.4266) ccw projected
  circle A1 centre (-91.2444, 95.4266) radius 4
  dimension "d6" = 8
  constraints: 1 centre point, 1 coincident
  measures "d6" diameter of A1
extrude "Kihúzás3" cut sketch "Vázlat2" against normal blind 10
chamfer "Letörés1" distance 0.4 angle 45 2 edges at (95.2444, 95.4266, 0) (95.2444, 95.4266, 10)
sketch "Vázlat3" plane through (0, 0, 10) normal (0, 0, 1) x (1, 0, 0)
  arc A0 (100.8284, 94.8732) -> (100.8284, 95.9801) centre (91.2444, 95.4266) ccw projected
  arc A1 (89.0351, 86.0843) -> (90.1252, 85.8921) centre (91.2444, 95.4266) ccw projected
  line L0 (90.2444, 92.8578) -> (92.2444, 92.8578)
  line L1 (92.2444, 92.8578) -> (92.2444, 90.5266)
  line L2 (92.2444, 90.5266) -> (90.2444, 90.5266)
  line L3 (90.2444, 90.5266) -> (90.2444, 92.8578)
  dimension "d12" = 2
  dimension "d13" = 1
  dimension "d14" = 4.9
  constraints: 8 end point, 2 parallel, 1 horizontal, 1 perpendicular
  measures "d12" distance of L1.end L2.end
  measures "d13" distance from line of L3 A1.centre
  measures "d14" distance from line of L2 A0.centre
extrude "Kihúzás4" cut sketch "Vázlat3" against normal blind 10
fillet "Lekerekítés3" radius 0.1 2 edges at (90.2444, 90.5266, 5) (92.2444, 90.5266, 5)
chamfer "Letörés2" distance 0.1 angle 45 2 edges at (92.2444, 91.5536, 5) (90.2444, 91.5536, 5)
sketch "Sketch4" plane through (0, 0, 10) normal (0, 0, 1) x (1, 0, 0)
  circle A0 centre (91.2444, 95.4864) radius 4.175
  point P0 (0, 0)
  dimension "d21" = 8.35
  constraints: 1 centre point
  measures "d21" diameter of A0
body "Solid1"
